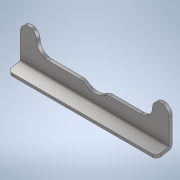
# Autodesk Inventor part: 補角片
Saved by Autodesk Inventor 2022 (Build 260153000, 153)
## iProperties
Created: 2022-03-10
Part Number: 補角片
Material: 不鏽鋼
Document SubType Name: Sheet Metal
Designer: 一條狗狗
Density: 8 g/cm^3
Appearance: 不鏽鋼 - 疏刷
Sheet Metal Rule: 預設 mm (_M)
Flat Pattern Width: 2.92287 cm
Flat Pattern Length: 9 cm
Flat Pattern Area: 26.3058 cm^2
Sheet Metal Width: 29.23 mm
Sheet Metal Length: 90.00 mm
Sheet Metal Area: 2630.58 mm^2
Author: 一條狗狗
Autodesk Inventor part; units mm, degrees
ref_plane "YZ Plane" through (0, 0, 0) normal (1, 0, 0) x (0, 1, 0)
ref_plane "XZ Plane" through (0, 0, 0) normal (0, 1, 0) x (-1, 0, 0)
ref_plane "XY Plane" through (0, 0, 0) normal (0, 0, 1) x (1, 0, 0)
sketch "草圖1" plane through (0, 0, 0) normal (0, 0, 1) x (1, 0, 0)
  line L0 (-163.791, 0) -> (203.4358, 0) projected
  line L1 (0, 6.9462) -> (0, -34.4284) projected
  line L2 (-40, 0) -> (-40, 0)
  line L3 (45, -5) -> (45, -25.5)
  line L4 (42.5, -28) -> (-42.5, -28)
  line L5 (-45, -25.5) -> (-45, -5)
  line L6 (-111.33, -20) -> (150.9748, -20)
  arc A0 (-45, -25.5) -> (-42.5, -28) centre (-42.5, -25.5) ccw
  arc A1 (42.5, -28) -> (45, -25.5) centre (42.5, -25.5) ccw
  line L7 (-35, -5) -> (-35, -5)
  line L8 (-28, -12) -> (-9, -12)
  line L9 (35, -5) -> (35, -5)
  line L10 (-35, 0) -> (35, 0) construction
  line L11 (40, 0) -> (40, 0)
  arc A2 (-40, 0) -> (-45, -5) centre (-40, -5) ccw
  arc A3 (45, -5) -> (40, 0) centre (40, -5) ccw
  arc A4 (-35, -5) -> (-40, 0) centre (-40, -5) ccw
  arc A5 (40, 0) -> (35, -5) centre (40, -5) ccw
  arc A6 (-35, -5) -> (-28, -12) centre (-28, -5) ccw
  arc A7 (28, -12) -> (35, -5) centre (28, -5) ccw
  circle A8 centre (-40, -5) radius 1.4
  circle A9 centre (40, -5) radius 1.4
  line L12 (-7.5, -12) -> (7.5, -12) construction
  line L13 (9, -12) -> (28, -12)
  line L14 (0, -18.0742) -> (0, 0) construction
  arc A10 (-6, -13) -> (6, -13) centre (0, -5) ccw
  arc A11 (-6, -13) -> (-9, -12) centre (-9, -17) ccw
  arc A12 (9, -12) -> (6, -13) centre (9, -17) ccw
  point P0 (-45, 0)
  point P1 (45, -28)
  point P2 (45, 0)
  point P3 (-45, -28)
  point P4 (-40, 0)
  point P5 (40, 0)
  point P6 (-7.1414, -12)
  point P7 (7.1414, -12)
  dimension "d0" = 90
  dimension "d1" = 8
  dimension "d2" = 20
  dimension "d6" = 2.5
  dimension "d7" = 5
  dimension "d8" = 5
  dimension "d9" = 8
  dimension "d10" = 10
  dimension "d11" = 7
  dimension "d12" = 2.8
  dimension "d19" = 5
  dimension "d20" = 5
  dimension "d21" = 10
  dimension "d22" = 15
  constraints: 28 end point, 24 point on circle, 24 tangent, 22 point on line, 13 centre point, 10 perpendicular, 5 equal radius, 4 horizontal, 4 parallel, 3 midpoint, 2 vertical alignment, 3 other
  measures "d0" distance between parallel lines of L3 L5
  measures "d1" distance between parallel lines of L4 L6
  measures "d2" distance between parallel lines of L2 L6
  measures "d6" radius of A0
  measures "d7" radius of A2
  measures "d8" radius of A4
  measures "d9" distance between parallel lines of L6 L8
  measures "d10" distance between parallel lines of L3 L9
  measures "d11" radius of A6
  measures "d12" diameter of A9
  measures "d19" distance edge to line of A10 L6
  measures "d20" radius of A11
  measures "d21" radius of A10
  measures "d22" distance from line of L6 A8.centre
extrude "平板1" add sketch "草圖1" against normal blind 2 contours A4 A6 L8 A11 A10 L1 L6 L5 A2 | A3 L3 L6 L1 A10 A12 L13 A7 A5 | L6 L1 L4 A0 L5 | L6 L3 A1 L4 L1 | A8 | A9
bend part "折彎零件1" radius 0.5 angle 80 line through (-111.33, -20, 0) along (1, 0, 0) centre toward (0, 0, 1) moving side (0, -1, 0) both sides no
sketch "草圖2" plane through (-45, -22.462, 0.0659) normal (0, -0.9848078, -0.1736482) x (1, 0, 0)
  line L0 (0, 0) -> (90, 0) projected
  line L1 (90, 4.8019) -> (90, 0) projected
  arc A0 (90, 4.8019) -> (87.5, 7.3019) centre (87.5, 4.8019) ccw projected
  line L2 (2.5, 7.3019) -> (87.5, 7.3019) projected
  arc A1 (2.5, 7.3019) -> (0, 4.8019) centre (2.5, 4.8019) ccw projected
  line L3 (0, 0) -> (0, 4.8019) projected
  line L4 (95.0452, 16.6838) -> (-5.2412, 16.6838)
  line L5 (-5.2412, 16.6838) -> (-5.2412, 5.3019)
  line L6 (-5.2412, 5.3019) -> (95.0452, 5.3019)
  line L7 (95.0452, 5.3019) -> (95.0452, 16.6838)
  point P0 (45, -3.9654)
  dimension "d23" = 2
  constraints: 8 end point, 2 parallel, 1 horizontal, 1 perpendicular
  measures "d23" distance between parallel lines of L2 L6
feature "手工切割" [suppressed]
equation "\"d24\" = 厚度"
equation "\"d3\" = 厚度"
equation "\"折彎半徑\" = 厚度"
equation "\"折彎離隙寬度\" = 厚度"
equation "\"折彎離隙深度\" = 0.5 * 厚度"
equation "\"轉角離隙大小\" = 4 * 厚度"
equation "\"最小剩餘\" = 2 * 厚度"
equation "\"轉移半徑\" = 折彎半徑"
equation "\"Jacobi半徑大小\" = 折彎半徑"
equation "\"間隙大小\" = 厚度"
equation "\"厚度\" = 2"
